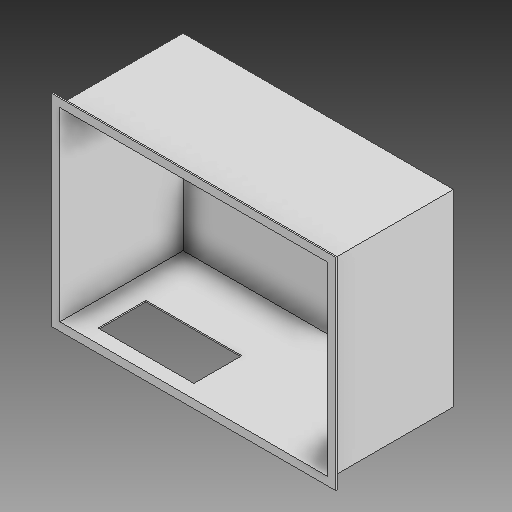
# Autodesk Inventor part: Schaltkasten
Saved by Autodesk Inventor 2021 (Build 250183000, 183)
## iProperties
Created: 2021-08-26
Part Number: Schaltkasten
Material: Generisch
Document SubType Name: Modeling
Designer: lukas
Density: 1 g/cm^3
Appearance: Vorgabe
Stock Number: Schaltkasten
Author: lukas
Autodesk Inventor part; units mm, degrees
ref_plane "YZ Plane" through (0, 0, 0) normal (1, 0, 0) x (0, 1, 0)
ref_plane "XZ Plane" through (0, 0, 0) normal (0, 1, 0) x (-1, 0, 0)
sketch "Skizze1" plane through (0, 0, 0) normal (0, 0, 1) x (1, 0, 0)
  line L0 (-276.5, 0) -> (276.5, 0) projected
  line L1 (0, -192.5) -> (0, 192.5) projected
  line L2 (-197.5, 137.5) -> (197.5, 137.5)
  line L3 (197.5, 137.5) -> (197.5, -137.5)
  line L4 (197.5, -137.5) -> (-197.5, -137.5)
  line L5 (-197.5, -137.5) -> (-197.5, 137.5)
  point P0 (0, 0)
  dimension "d0" = 395
  dimension "d1" = 275
  constraints: 8 end point, 2 parallel, 1 horizontal, 1 perpendicular, 2 other
  measures "d0" distance between parallel lines of L3 L5
  measures "d1" distance between parallel lines of L2 L4
extrude "Extrusion1" add sketch "Skizze1" along normal blind 180
sketch "Skizze2" plane through (0, 0, 180) normal (0, 0, 1) x (1, 0, 0)
  line L0 (-195.5, 135.5) -> (195.5, 135.5)
  line L1 (195.5, 135.5) -> (195.5, -135.5)
  line L2 (195.5, -135.5) -> (-195.5, -135.5)
  line L3 (-195.5, -135.5) -> (-195.5, 135.5)
  line L4 (197.5, 137.5) -> (-197.5, 137.5) projected
  line L5 (197.5, -137.5) -> (197.5, 137.5) projected
  line L6 (-197.5, -137.5) -> (197.5, -137.5) projected
  line L7 (-197.5, 137.5) -> (-197.5, -137.5) projected
  point P0 (0, 0)
  dimension "d4" = 2
  dimension "d5" = 2
  dimension "d6" = 2
  dimension "d7" = 2
  constraints: 8 end point, 2 parallel, 1 horizontal, 1 perpendicular
  measures "d4" distance between parallel lines of L4 L0
  measures "d5" distance between parallel lines of L5 L1
  measures "d6" distance between parallel lines of L6 L2
  measures "d7" distance between parallel lines of L7 L3
extrude "Extrusion2" cut sketch "Skizze2" against normal blind 178 contours L0 L1 L2 L3
ref_plane "Arbeitsebene1" through (0, 0, 180) normal (0, 0, 1) x (1, 0, 0)
sketch "Skizze4" plane through (0, 0, 180) normal (0, 0, 1) x (1, 0, 0)
  line L0 (-207.5, -147.5) -> (207.5, -147.5)
  line L1 (207.5, -147.5) -> (207.5, 147.5)
  line L2 (207.5, 147.5) -> (-207.5, 147.5)
  line L3 (-207.5, 147.5) -> (-207.5, -147.5)
  line L4 (-195.5, -135.5) -> (-195.5, 135.5) projected
  line L5 (-195.5, 135.5) -> (195.5, 135.5) projected
  line L6 (195.5, 135.5) -> (195.5, -135.5) projected
  line L7 (195.5, -135.5) -> (-195.5, -135.5) projected
  point P0 (0, 0)
  dimension "d17" = 12
  dimension "d18" = 12
  dimension "d19" = 12
  dimension "d20" = 12
  constraints: 8 end point, 2 parallel, 1 horizontal, 1 perpendicular
  measures "d17" distance between parallel lines of L4 L3
  measures "d18" distance between parallel lines of L2 L5
  measures "d19" distance between parallel lines of L1 L6
  measures "d20" distance between parallel lines of L7 L0
extrude "Extrusion4" add sketch "Skizze4" along normal blind 2
sketch "Skizze5" plane through (0, 0, 0) normal (0, 0, -1) x (-1, 0, 0)
  line L0 (-197.5, -137.5) -> (-197.5, 137.5) projected
  line L1 (-197.5, 137.5) -> (197.5, 137.5) projected
  circle A0 centre (-147.5, 87.5) radius 15
  point P0 (0, 0)
  dimension "d23" = 50
  dimension "d24" = 50
  dimension "d25" = 30
  constraints: 1 centre point, 1 coincident
  measures "d23" distance from line of point (-147.5, 87.5) L0
  measures "d24" distance from line of point (-147.5, 87.5) L1
  measures "d25" diameter of A0
extrude "Extrusion5" cut sketch "Skizze5" against normal blind 10
sketch "Skizze6" plane through (-195.5, -135.5, 2) normal (0, 1, 0) x (1, 0, 0)
  line L0 (35.8194, -90) -> (175.8194, -90)
  line L1 (175.8194, -90) -> (175.8194, -160)
  line L2 (175.8194, -160) -> (35.8194, -160)
  line L3 (35.8194, -160) -> (35.8194, -90)
  line L4 (391, -180) -> (0, -180) projected
  point P0 (195.5, 2)
  dimension "d28" = 70
  dimension "d29" = 140
  dimension "d30" = 20
  constraints: 8 end point, 2 parallel, 1 horizontal, 1 perpendicular
  measures "d28" distance between parallel lines of L0 L2
  measures "d29" distance between parallel lines of L1 L3
  measures "d30" distance between parallel lines of L2 L4
extrude "Extrusion6" cut sketch "Skizze6" against normal blind 10
sketch "Skizze7" plane through (0, 0, 2) normal (0, 0, 1) x (1, 0, 0)
  line L0 (-195.5, -135.5) -> (-195.5, 135.5) projected
  line L1 (-195.5, 135.5) -> (195.5, 135.5) projected
  circle A0 centre (-165.5, 105.5) radius 7.5
  point P0 (0, 0)
  dimension "d33" = 30
  dimension "d34" = 30
  dimension "d35" = 15
  constraints: 1 centre point, 1 coincident
  measures "d33" distance from line of point (-165.5, 105.5) L0
  measures "d34" distance from line of L1 point (-165.5, 105.5)
  measures "d35" diameter of A0
extrude "Extrusion7" cut sketch "Skizze7" against normal blind 10
sketch "Skizze8" plane through (-195.5, -135.5, 2) normal (0, 1, 0) x (1, 0, 0)
  line L0 (391, 0) -> (0, 0) projected
  line L1 (391, 0) -> (391, -180) projected
  circle A0 centre (361, -40) radius 5
  circle A1 centre (331, -40) radius 5
  point P0 (195.5, 2)
  dimension "d38" = 40
  dimension "d39" = 40
  dimension "d40" = 30
  dimension "d41" = 30
  dimension "d42" = 10
  dimension "d43" = 10
  constraints: 2 centre point, 2 coincident
  measures "d38" distance from line of point (361, -40) L0
  measures "d39" distance from line of L0 point (331, -40)
  measures "d40" distance from line of point (361, -40) L1
  measures "d41" distance of point (361, -40) point (331, -40)
  measures "d42" diameter of A0
  measures "d43" diameter of A1
extrude "Extrusion8" cut sketch "Skizze8" against normal blind 10
